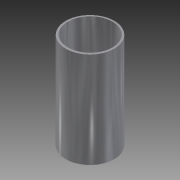
# Autodesk Inventor part: Inner Cup
Saved by Autodesk Inventor 2014 (Build 180170000, 170)
## iProperties
Created: 2014-06-10
Part Number: Inner Cup
Material: Generic
Document SubType Name: Modeling
Designer: Nabeel
Density: 1 g/cm^3
Appearance: Default
Author: Nabeel
Autodesk Inventor part; units mm, degrees
ref_plane "YZ Plane" through (0, 0, 0) normal (1, 0, 0) x (0, 1, 0)
ref_plane "XZ Plane" through (0, 0, 0) normal (0, 1, 0) x (-1, 0, 0)
ref_plane "XY Plane" through (0, 0, 0) normal (0, 0, 1) x (1, 0, 0)
sketch "Sketch1" plane through (0, 0, 0) normal (0, 0, 1) x (1, 0, 0)
  line L0 (-26.6, 0) -> (26.6, 0) projected
  line L1 (0, -26.6) -> (0, 26.6) projected
  circle A0 centre (0, 0) radius 19
  dimension "d0" = 38
  constraints: 1 centre point, 1 coincident
  measures "d0" diameter of A0
extrude "Extrusion1" add sketch "Sketch1" along normal blind 75
hole "Hole2" at (-0.0824, 0.2472, 75) direction (0, 0, -1) diameter 35 depth 71
body "Solid1"
